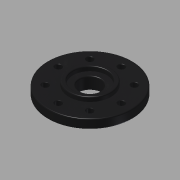
# Autodesk Inventor part: bottom-arm
Saved by Autodesk Inventor 2016 (Build 200138000, 138)
## iProperties
Created: 2013-07-13
Part Number: bottom-arm
Material: PET Plastic
Document SubType Name: Modeling
Designer: Maurice
Density: 1.541 g/cm^3
Appearance: Polycarbonate - Clear
Mass: 1.05043 g
Surface Area: 8.80051 cm^2
Volume: 0.681653 cm^3
Author: Maurice
Autodesk Inventor part; units mm, degrees
ref_plane "YZ Plane" through (0, 0, 0) normal (1, 0, 0) x (0, 1, 0)
ref_plane "XZ Plane" through (0, 0, 0) normal (0, 1, 0) x (-1, 0, 0)
ref_plane "XY Plane" through (0, 0, 0) normal (0, 0, 1) x (1, 0, 0)
sketch "Sketch1" plane through (0, 0, 0) normal (0, 1, 0) x (-1, 0, 0)
  circle A0 centre (0, 0) radius 10
  dimension "d0" = 20
  constraints: 1 centre point, 1 coincident
  measures "d0" diameter of A0
extrude "Extrusion1" add sketch "Sketch1" along normal blind 2.14
sketch "Sketch2" plane through (0, 2.14, 0) normal (0, 1, 0) x (1, 0, 0)
  circle A0 centre (0, 0) radius 10 projected
  circle A1 centre (0, 0) radius 5
  dimension "d3" = 10
  constraints: 1 centre point, 1 coincident
  measures "d3" diameter of A1
extrude "Extrusion2" add sketch "Sketch2" along normal blind 1 contours A1
sketch "Sketch3" plane through (0, 0, 0) normal (0, -1, 0) x (1, 0, 0)
  circle A0 centre (0, 0) radius 10 projected
  circle A1 centre (0, 0) radius 5
  dimension "d6" = 10
  constraints: 1 centre point, 1 coincident
  measures "d6" diameter of A1
extrude "Extrusion3" add sketch "Sketch3" along normal blind 1 contours A1
hole "Hole1" at (0, 3.14, 0) direction (0, -1, 0) diameter 5 end through all
sketch "Sketch4" plane through (0, 3.14, 0) normal (0, 1, 0) x (1, 0, 0)
  circle A0 centre (0, 0) radius 2.5 projected
  circle A1 centre (0, 0) radius 5 projected
  circle A2 centre (0, 0) radius 4
  dimension "d18" = 8
  constraints: 1 centre point, 1 coincident
  measures "d18" diameter of A2
extrude "Extrusion4" cut sketch "Sketch4" against normal blind 1 contours A2
sketch "Sketch5" plane through (0, 2.14, 0) normal (0, 1, 0) x (1, 0, 0)
  circle A0 centre (0, 0) radius 5 projected
  circle A1 centre (0, 0) radius 10 projected
  point P0 (0, 7.5)
  point P1 (-5.3033, 5.3033)
  point P2 (-7.5, 0)
  point P3 (-5.3033, -5.3033)
  point P4 (0, -7.5)
  point P5 (5.3033, -5.3033)
  point P6 (7.5, 0)
  point P7 (5.3033, 5.3033)
  dimension "d21" = 5
  dimension "d22" = 7.5
  dimension "d25" = 360
  constraints: 1 vertical alignment, 9 other
  measures "d21" radial gap between concentric circles of A1 A0
  measures "d22" distance of A0.centre point (0, 7.5)
hole "Hole2" at (0, 2.14, -7.5) at (-5.3033, 2.14, -5.3033) at (-7.5, 2.14, 0) at (-5.3033, 2.14, 5.3033) at (0, 2.14, 7.5) at (5.3033, 2.14, 5.3033) at (7.5, 2.14, 0) at (5.3033, 2.14, -5.3033) direction (0, -1, 0) diameter 1.5 end through all
chamfer "Chamfer1" distance 0.5 angle 45 1 edges at (0, -1, -2.5)
fillet "Fillet1" radius 0.25 6 edges at (10, 0, 0) (10, 2.14, 0) (-5, -1, 0) (-5, 3.14, 0) (-4, 3.14, 0) (0, 2.14, -2.5)
chamfer "Chamfer2" distance 0.1 angle 45 16 edges at (5.3033, 0, -6.0533) (0, 0, -8.25) (-5.3033, 0, -6.0533) (7.5, 0, -0.75) (5.3033, 0, 4.5533) (-7.5, 0, -0.75) (0, 0, 6.75) (-5.3033, 0, 4.5533) (5.3033, 2.14, -6.0533) (0, 2.14, -8.25) (-5.3033, 2.14, -6.0533) (7.5, 2.14, -0.75) (5.3033, 2.14, 4.5533) (-7.5, 2.14, -0.75) (0, 2.14, 6.75) (-5.3033, 2.14, 4.5533)
body "Solid1"
